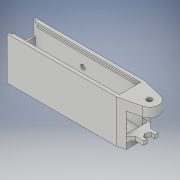
# Autodesk Inventor part: LampeSolaire2_Casing 3D printed
Saved by Autodesk Inventor 2019 (Build 230136000, 136)
## iProperties
Created: 2020-09-21
Part Number: LampeSolaire2_Casing 3D printed
Material: Generic
Document SubType Name: Modeling
Designer: nicolas
Density: 1 g/cm^3
Appearance: Default
Mass: 36.8708 g
Surface Area: 353.111 cm^2
Volume: 36.8708 cm^3
Author: nicolas
## iProperties of the stored document LampeSolaire2_Casing_3DPrint.ipt
Created: 2020-10-22
Part Number: LampeSolaire2_Casing_3DPrint
Material: Generic
Document SubType Name: Modeling
Designer: nicolas
Density: 1 g/cm^3
Appearance: Default
Author: nicolas
Autodesk Inventor part; units mm, degrees
ref_plane "XZ Plane" through (0, 0, 0) normal (0, 1, 0) x (-1, 0, 0)
ref_plane "XY Plane" through (0, 0, 0) normal (0, 0, 1) x (1, 0, 0)
sketch "Sketch5" plane through (0, 0, 0) normal (0, 1, 0) x (-1, 0, 0)
  line L0 (0, 12.5) -> (-110, 12.5)
  line L1 (-110, -12.5) -> (0, -12.5)
  arc A0 (-131.7462, 7.2939) -> (-131.7462, -7.2939) centre (-130, 0) ccw
  line L2 (-131.7462, -7.2939) -> (-110, -12.5)
  line L3 (-131.7462, 7.2939) -> (-110, 12.5)
  circle A1 centre (-130, 0) radius 2.75
  line L4 (0, -12.5) -> (0, 0)
  line L5 (0, 0) -> (0, 12.5)
  line L6 (-110, -12.5) -> (-110, 0) construction
  line L7 (-110, 0) -> (-110, 12.5) construction
  line L8 (-110, 0) -> (0, 0) construction
  point P0 (0, 0)
  dimension "d52" = 15
  dimension "d53" = 20
  dimension "d54" = 5.5
  dimension "d55" = 110
  dimension "d56" = 25
  constraints: 18 end point, 5 equal length, 3 vertical, 2 centre point, 2 point on circle, 2 point on line, 2 tangent, 1 coincident, 1 horizontal
  measures "d52" diameter of A0
  measures "d53" horizontal distance of L1.start A0.centre
  measures "d54" diameter of A1
  measures "d55" distance of L1.start L1.end
  measures "d56" distance of L1.end L0.start
sketch "Sketch6" plane through (0, 0, 0) normal (0, 0, 1) x (1, 0, 0)
  line L0 (0, -21) -> (0, 21)
  point P0 (0, 0)
  point P1 (0, 0)
  dimension "d25" = 42
  constraints: 2 end point, 1 coincident, 1 midpoint, 1 vertical
  measures "d25" distance of L0.start L0.end
sweep "Sweep1" add profiles "Sketch5" path "Sketch6" contours L5 L4 L1 L2 A0 L3 L0 | A1
shell "Shell1" thickness 2 outward yes removed faces 1 at (73.3333, 21, 0)
sketch "Sketch12" plane through (0, -21, 12.5) normal (0, 1, 0) x (1, 0, 0)
  line L0 (0, 12.5) -> (10, 12.5) construction
  line L1 (10, 12.5) -> (98, 12.5) construction
  line L2 (0, 0) -> (0, 25) projected
  point P0 (0, 12.5)
  dimension "d58" = 88
  dimension "d59" = 10
  constraints: 4 end point, 4 midpoint, 2 coincident, 2 point on line, 1 horizontal
  measures "d58" distance of L0.end L1.end
  measures "d59" distance of L0.start L0.end
hole "Hole4" at (10, -21, 0) at (98, -21, 0) direction (0, -1, 0) diameter 5.5 depth 2 tip angle 118
sketch "Sketch14" plane through (0, -21, 12.5) normal (0, 1, 0) x (1, 0, 0)
  arc A0 (131.7462, 5.2061) -> (131.7462, 19.7939) centre (130, 12.5) ccw projected
  circle A1 centre (130, 12.5) radius 2.75
  circle A2 centre (130, 12.5) radius 9.5
  point P0 (0, 12.5)
  dimension "d67" = 5.5
  dimension "d68" = 19
  constraints: 2 centre point, 2 coincident
  measures "d67" diameter of A1
  measures "d68" diameter of A2
extrude "Extrusion4" add sketch "Sketch14" along normal up to surface (42 mm away)
sketch "Sketch15" plane through (130, -21, 0) normal (0, 1, 0) x (1, 0, 0)
  circle A0 centre (0, 0) radius 2.75 projected
  point P0 (-130, 0)
extrude "Extrusion5" cut sketch "Sketch15" against normal up to next
ref_plane "Work Plane4" through (139.5, -21, 0) normal (1, 0, 0) x (0, 1, 0)
sketch "Sketch16" plane through (139.5, -21, 0) normal (1, 0, 0) x (0, 1, 0)
  line L0 (32.35, 12.5) -> (9.65, 12.5)
  line L1 (9.65, 12.5) -> (9.65, -12.5)
  line L2 (9.65, -12.5) -> (32.35, -12.5)
  line L3 (32.35, -12.5) -> (32.35, 12.5)
  line L4 (32.35, 12.5) -> (9.65, -12.5) construction
  line L5 (9.65, 12.5) -> (32.35, -12.5) construction
  point P0 (21, 0)
  dimension "d73" = 22.7
  dimension "d74" = 25
  constraints: 12 end point, 2 midpoint, 2 parallel, 1 horizontal, 1 perpendicular
  measures "d73" distance of L2.end L1.end
  measures "d74" distance of L1.end L0.end
extrude "Extrusion6" cut sketch "Sketch16" against normal up to next
sketch "Sketch17" plane through (-2, -23, 14.5) normal (0, -1, 0) x (1, 0, 0)
  circle A0 centre (132, -14.5) radius 2.75 projected
  circle A1 centre (132, -14.5) radius 4 construction
  line L0 (134.3094, -10.5) -> (136.6188, -14.5)
  line L1 (136.6188, -14.5) -> (134.3094, -18.5)
  line L2 (134.3094, -10.5) -> (129.6906, -10.5)
  line L3 (129.6906, -10.5) -> (127.3812, -14.5)
  line L4 (127.3812, -14.5) -> (129.6906, -18.5)
  line L5 (129.6906, -18.5) -> (134.3094, -18.5)
  point P0 (2, -14.5)
  dimension "d77" = 8
  constraints: 12 end point, 6 tangent, 4 equal length, 2 horizontal, 1 centre point, 1 coincident
  measures "d77" diameter of A1
extrude "Extrusion7" cut sketch "Sketch17" against normal blind 4
sketch "Sketch22" plane through (0, -21, 12.5) normal (0, 1, 0) x (1, 0, 0)
  circle A0 centre (98, 12.5) radius 2.75 projected
  circle A1 centre (98, 12.5) radius 6
  circle A2 centre (10, 12.5) radius 2.75 projected
  circle A3 centre (10, 12.5) radius 6
  point P0 (0, 12.5)
  dimension "d96" = 12
  dimension "d97" = 12
  constraints: 2 centre point, 2 coincident
  measures "d96" diameter of A1
  measures "d97" diameter of A3
extrude "Extrusion12" add sketch "Sketch22" along normal blind 4
sketch "Sketch21" plane through (-2, -23, 14.5) normal (0, -1, 0) x (1, 0, 0)
  circle A0 centre (12, -14.5) radius 2.75 projected
  circle A1 centre (100, -14.5) radius 2.75 projected
  circle A2 centre (12, -14.5) radius 4 construction
  line L0 (8, -16.8094) -> (8, -12.1906)
  line L1 (8, -12.1906) -> (12, -9.8812)
  line L2 (12, -9.8812) -> (16, -12.1906)
  line L3 (16, -12.1906) -> (16, -16.8094)
  line L4 (16, -16.8094) -> (12, -19.1188)
  line L5 (12, -19.1188) -> (8, -16.8094)
  line L6 (96, -16.8094) -> (96, -12.1906)
  line L7 (96, -12.1906) -> (100, -9.8812)
  line L8 (100, -9.8812) -> (104, -12.1906)
  line L9 (104, -12.1906) -> (104, -16.8094)
  line L10 (104, -16.8094) -> (100, -19.1188)
  line L11 (100, -19.1188) -> (96, -16.8094)
  circle A3 centre (100, -14.5) radius 4 construction
  point P0 (2, -14.5)
  dimension "d92" = 8
  dimension "d93" = 8
  constraints: 24 end point, 4 coincident, 2 centre point, 2 tangent, 2 vertical, 26 other
  measures "d92" diameter of A2
  measures "d93" diameter of A3
extrude "Extrusion11" cut sketch "Sketch21" against normal blind 4
sketch "Sketch20" plane through (-2, 21, -14.5) normal (0, 1, 0) x (1, 0, 0)
  line L0 (128.0755, -23.1515) -> (112, -27) projected
  arc A0 (128.0755, -23.1515) -> (128.0755, -5.8485) centre (132, -14.5) ccw projected
  line L1 (112, -2) -> (128.0755, -5.8485) projected
  line L2 (112, -27) -> (112, -2)
  circle A1 centre (132, -14.5) radius 2.75 projected
  constraints: 2 end point, 1 vertical
extrude "Extrusion10" add sketch "Sketch20" against normal blind 2
ref_plane "Work Plane5" through (110, 21, 0) normal (0, 0, -1) x (-1, 0, 0)
sketch "Sketch25" plane through (110, -21, 12.5) normal (0, 0, -1) x (-1, 0, 0)
  line L0 (0, 42) -> (109.25, 42)
  line L1 (110, 42) -> (110, 40.5) construction
  line L2 (110, 40.5) -> (108.5, 40.5) construction
  line L3 (0, 40.5) -> (0, 42)
  line L4 (0, 42) -> (110, 42) projected
  line L5 (0, 39) -> (106.5, 39)
  line L6 (110, 39) -> (110, 37.5) construction
  line L7 (110, 37.5) -> (108, 37.5) construction
  line L8 (0, 37.5) -> (0, 39)
  line L9 (0, 32.35) -> (0, 40) projected
  line L10 (0, 40) -> (0, 42) projected
  line L11 (110, 0) -> (110, 42) projected
  line L12 (0, 40.5) -> (1.5, 40.5)
  line L13 (1.5, 40.5) -> (1.5, 39)
  line L14 (1.5, 39) -> (0, 39)
  line L15 (0, 39) -> (0, 40.5)
  line L16 (108, 37.5) -> (107.25, 38.25) construction
  line L17 (110, 42) -> (109.25, 41.25) construction
  line L18 (108.5, 40.5) -> (1.5, 40.5)
  line L19 (106.5, 39) -> (110, 39) construction
  line L20 (108, 37.5) -> (107.25, 37.5) construction
  line L21 (107.25, 37.5) -> (107.25, 38.25)
  line L22 (107.25, 37.5) -> (0, 37.5)
  line L23 (107.25, 38.25) -> (106.5, 39)
  line L24 (109.25, 41.25) -> (109.25, 42)
  line L25 (110, 42) -> (0, 42) construction
  line L26 (109.25, 41.25) -> (108.5, 40.5)
  line L27 (109.25, 42) -> (110, 42) construction
  point P0 (110, 21)
  point P1 (107.25, 37.875)
  dimension "d105" = 1.5
  dimension "d106" = 1.5
  dimension "d107" = 1.5
  dimension "d110" = 1.5
  dimension "d111" = 1.5
  dimension "d132" = 45
  dimension "d133" = 45
  dimension "d134" = 2
  dimension "d138" = 0.75
  dimension "d139" = 0.75
  constraints: 46 end point, 14 parallel, 6 collinear, 6 perpendicular, 5 horizontal, 1 midpoint, 1 point on line, 1 vertical
  measures "d105" distance of L1.start L1.end
  measures "d106" distance of L6.start L6.end
  measures "d107" distance between parallel lines of L2 L5
  measures "d110" distance of L13.end L14.end
  measures "d111" distance of L12.end L13.end
  measures "d132" angle of L0 L17
  measures "d133" angle of L7 L16
  measures "d134" distance from line of L6 L7.end
  measures "d138" distance of L20.end L7.end
  measures "d139" distance of L1.start L0.end
extrude "Extrusion15" add sketch "Sketch25" along normal blind 1.5
mirror "Mirror1" about plane through (0, 0, 0) normal (0, 0, 1) of "Extrusion15"
sketch "Sketch26" plane through (0, -21, 12.5) normal (1, 0, 0) x (0, 0, -1)
  line L0 (0, 42) -> (25, 42) projected
  line L1 (0, 0) -> (0, 42) projected
  line L2 (25, 0) -> (0, 0) projected
  line L3 (25, 0) -> (25, 42) projected
  line L4 (0, 27) -> (25, 27)
  line L5 (25, 27) -> (0, 27)
  line L6 (0, 27) -> (0, 42)
  line L7 (0, 42) -> (25, 42)
  line L8 (25, 42) -> (25, 27)
  point P0 (12.5, 21)
  dimension "d112" = 15
  constraints: 10 end point, 2 horizontal, 2 parallel, 1 perpendicular, 1 point on line
  measures "d112" distance between parallel lines of L0 L4
extrude "Extrusion16" cut sketch "Sketch26" against normal up to next contours L0 L3 L4 L1
sketch "Sketch29" plane through (-2, -23, -14.5) normal (-1, 0, 0) x (0, 0, 1)
  circle A0 centre (11.5, 22) radius 1.5
  line L0 (18.5, 0) -> (14.5, 0) projected
  circle A1 centre (17.5, 22) radius 1.5
  line L1 (14.5, 0) -> (14.5, 4) projected
  line L2 (14.5, 0) -> (14.5, 29) construction
  line L3 (11.5, 22) -> (14.5, 22)
  line L4 (17.5, 22) -> (14.5, 22)
  line L5 (27, 29) -> (2, 29) projected
  point P0 (14.5, 23)
  dimension "d123" = 3
  dimension "d125" = 3
  dimension "d127" = 3
  dimension "d136" = 7
  constraints: 6 end point, 2 centre point, 2 collinear, 1 horizontal, 1 midpoint, 1 point on line
  measures "d123" diameter of A0
  measures "d125" diameter of A1
  measures "d127" distance of L3.start L3.end
  measures "d136" distance between parallel lines of L5 L3
extrude "Extrusion19" cut sketch "Sketch29" against normal up to next
sketch "Sketch36" plane through (110, -11.35, 12.5) normal (0, 1, 0) x (1, 0, 0)
  line L0 (8.5902, 25) -> (22.2118, 21.7389) projected
  line L1 (22.2118, 3.2611) -> (8.5902, 0) projected
  line L2 (8.5902, 25) -> (8.5902, 0)
  arc A0 (22.2118, 3.2611) -> (22.2118, 21.7389) centre (20, 12.5) ccw projected
  point P0 (-110, 12.5)
  constraints: 2 end point, 1 vertical
extrude "Extrusion24" cut sketch "Sketch36" against normal through all
sketch "Sketch37" plane through (0, -21, -12.5) normal (0, 1, 0) x (1, 0, 0)
  line L0 (118.5902, -22.9435) -> (118.5902, -2.0565) projected
  line L1 (118.5902, -2.0565) -> (118.5902, -22.9435)
  line L2 (118.5902, -2.0565) -> (116.6451, -1.5909)
  line L3 (118.5902, -2.0565) -> (110, 0) projected
  line L4 (116.6451, -1.5909) -> (116.6451, -23.4091)
  line L5 (110, -25) -> (118.5902, -22.9435) projected
  point P0 (0, -12.5)
  dimension "d151" = 2
  constraints: 6 end point, 2 point on line, 1 collinear, 1 parallel
  measures "d151" distance of L0.end L2.end
extrude "Extrusion25" add sketch "Sketch37" along normal up to surface (9.65 mm away)
sketch "Sketch38" plane through (118.5902, -11.35, 12.5) normal (1, 0, 0) x (0, 0, -1)
  line L0 (0, 0) -> (25, 0) projected
  line L1 (20, -4) -> (20, 0)
  line L2 (20, 0) -> (5, 0)
  line L3 (5, 0) -> (5, -4)
  line L4 (5, -4) -> (20, -4)
  line L5 (20, -4) -> (5, 0) construction
  line L6 (20, 0) -> (5, -4) construction
  line L7 (0, 0) -> (25, -11.65) construction
  line L8 (27, -11.65) -> (-2, -11.65) projected
  line L9 (25, 0) -> (0, -11.65) construction
  line L10 (12.5, -5.825) -> (12.5, 0) construction
  point P0 (12.5, 11.35)
  point P1 (12.5, -2)
  point P2 (12.5, -2)
  dimension "d154" = 15
  dimension "d157" = 4
  constraints: 18 end point, 6 midpoint, 2 parallel, 2 perpendicular, 2 point on line, 1 collinear
  measures "d154" distance of L2.end L1.end
  measures "d157" distance of L1.start L1.end
extrude "Extrusion26" add sketch "Sketch38" along normal blind 13
sketch "Sketch39" plane through (110, -11.35, -12.5) normal (0, 1, 0) x (1, 0, 0)
  circle A0 centre (20, -12.5) radius 2.75 projected
  line L0 (17.6906, -8.5) -> (22.3094, -8.5)
  line L1 (22.3094, -8.5) -> (24.6188, -12.5)
  line L2 (24.6188, -12.5) -> (22.3094, -16.5)
  line L3 (22.3094, -16.5) -> (17.6906, -16.5)
  line L4 (17.6906, -16.5) -> (15.3812, -12.5)
  line L5 (15.3812, -12.5) -> (17.6906, -8.5)
  circle A1 centre (20, -12.5) radius 4 construction
  point P0 (-110, -12.5)
  dimension "d158" = 8
  constraints: 12 end point, 2 coincident, 1 centre point, 1 horizontal, 1 tangent, 13 other
  measures "d158" diameter of A1
extrude "Extrusion27" cut sketch "Sketch39" against normal up to next contours A0 | L0 L1 L2 L3 L4 L5
chamfer "Chamfer1" distance 5 angle 45 2 edges at (118.5902, -13.35, -7.5) (118.5902, -13.35, 7.5)
chamfer "Chamfer2" distance 2 angle 45 3 edges at (118.5902, -15.35, -10) (118.5902, -15.35, 0) (118.5902, -15.35, 9.9999)
sketch "Sketch40" plane through (110, 11.35, -12.5) normal (0, -1, 0) x (1, 0, 0)
  circle A0 centre (20, 12.5) radius 2.75 projected
  circle A1 centre (20, 12.5) radius 4.275
  point P0 (-110, 12.5)
  dimension "d167" = 8.55
  constraints: 1 centre point, 1 coincident
  measures "d167" diameter of A1
extrude "Extrusion28" cut sketch "Sketch40" against normal blind 0.1
sketch "Sketch41" plane through (110.2361, -23, -14.5) normal (0, 0, -1) x (-1, 0, 0)
  line L0 (0, 0) -> (112.2361, 0) projected
  line L1 (112.2361, 0) -> (112.2361, 44) projected
  circle A0 centre (61.2361, 26.35) radius 2.5
  line L2 (0, 44) -> (112.2361, 44) projected
  point P0 (110.2361, 23)
  dimension "d176" = 51
  dimension "d177" = 5
  dimension "d179" = 17.65
  constraints: 1 centre point
  measures "d176" distance from line of A0.centre L1
  measures "d177" diameter of A0
  measures "d179" distance from line of L2 A0.centre
extrude "Extrusion29" cut sketch "Sketch41" against normal up to next
body "Solid2"
